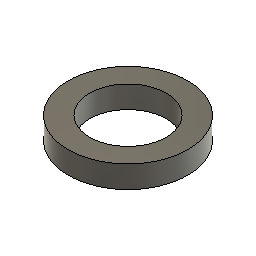
cone set sample (Autodesk Fusion 360 design; units mm, degrees)
part number: 2025-04-22-15-12-20-019
Autodesk Fusion 360 part; units mm, degrees
sketch "Sketch1" plane through (0, 0, 0) normal (0, 1, 0) x (1, 0, 0)
  circle A0 centre (0, 0) radius 28.45
  circle A1 centre (0, 0) radius 44.45
  dimension "d1" = 56.9
  dimension "d2" = 88.9
  constraint coincident A0.centre A1.centre
  constraint concentric A0 A1
  measures "d1" diameter of A0
  measures "d2" diameter of A1
extrude "Extrude1" add sketch "Sketch1" along normal blind 16.5
